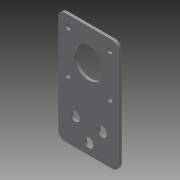
# Autodesk Inventor part: Part4
Saved by Autodesk Inventor 2015 SP1 (Build 190203100, 203)
## iProperties
Created: 2015-03-28
Part Number: Part4
Material: Generic
Document SubType Name: Modeling
Designer: Cyril
Density: 1 g/cm^3
Appearance: Default
Author: Cyril
Autodesk Inventor part; units mm, degrees
ref_plane "YZ Plane" through (0, 0, 0) normal (1, 0, 0) x (0, 1, 0)
ref_plane "XZ Plane" through (0, 0, 0) normal (0, 1, 0) x (-1, 0, 0)
ref_plane "XY Plane" through (0, 0, 0) normal (0, 0, 1) x (1, 0, 0)
sketch "Sketch1" plane through (0, 0, 0) normal (0, 0, 1) x (1, 0, 0)
  circle A0 centre (0, 0) radius 11
  line L0 (0, 0) -> (0, 0) construction
  circle A1 centre (-10, -39) radius 3.5
  circle A2 centre (10, -39) radius 3.5
  circle A3 centre (0, -51) radius 3.5
  line L1 (0, 0) -> (0, -50) construction
  circle A4 centre (15.5, 15.5) radius 2
  circle A5 centre (-15.5, 15.5) radius 2
  circle A6 centre (-15.5, -15.5) radius 2
  circle A7 centre (15.5, -15.5) radius 2
  line L2 (0, 0) -> (-11, 0) construction
  line L3 (-10, -39) -> (10, -39) construction
  line L4 (-17.5, 23.5) -> (17.5, 23.5)
  arc A8 (22.5, 18.5) -> (17.5, 23.5) centre (17.5, 18.5) ccw
  line L5 (22.5, 18.5) -> (22.5, -54)
  arc A9 (17.5, -59) -> (22.5, -54) centre (17.5, -54) ccw
  line L6 (17.5, -59) -> (-17.5, -59)
  arc A10 (-22.5, -54) -> (-17.5, -59) centre (-17.5, -54) ccw
  line L7 (-22.5, -54) -> (-22.5, 18.5)
  arc A11 (-17.5, 23.5) -> (-22.5, 18.5) centre (-17.5, 18.5) ccw
  dimension "d0" = 22
  dimension "d39" = 7
  dimension "d40" = 20
  dimension "d42" = 39
  dimension "d44" = 4
  dimension "d45" = 31
  dimension "d46" = 31
  dimension "d51" = 12
  dimension "d52" = 45
  dimension "d53" = 8
  dimension "d54" = 5
  dimension "d55" = 8
  constraints: 16 end point, 11 centre point, 8 point on circle, 8 tangent, 5 equal radius, 3 horizontal, 3 perpendicular, 2 coincident, 1 horizontal alignment, 1 point on line, 1 vertical, 7 other
  measures "d39" diameter of A1
  measures "d40" distance of L3.end L3.start
  measures "d42" vertical distance of L0.start L3.start
  measures "d44" diameter of A4
  measures "d45" distance of A7.centre A4.centre
  measures "d46" distance of A5.centre A4.centre
  measures "d51" distance from line of A3.centre L3
  measures "d52" distance between parallel lines of L5 L7
  measures "d53" distance from line of A5.centre L4
  measures "d54" radius of A11
  measures "d55" distance from line of L6 A3.centre
extrude "Extrusion4" add sketch "Sketch1" along normal blind 2
equation "\"d46\" = d45"
body "Solid2"
